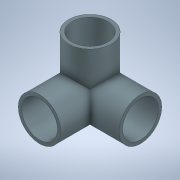
# Autodesk Inventor part: hoek drieweg
Saved by Autodesk Inventor 2020.2 (Build 242310000, 310)
## iProperties
Created: 2019-11-27
Part Number: hoek drieweg
Material: ABS Plastic
Document SubType Name: Modeling
Designer: Gebruiker
Density: 1.06 g/cm^3
Appearance: Lead
Author: Gebruiker
Autodesk Inventor part; units mm, degrees
sketch "Sketch1" plane through (0, 0, 0) normal (0, 1, 0) x (-1, 0, 0)
  line L0 (0, 0) -> (0, 30)
  line L1 (0, 0) -> (-30, 0)
  dimension "d0" = 30
  dimension "d1" = 30
  constraints: 4 end point, 1 horizontal, 1 vertical
  measures "d0" distance of L0.start L0.end
  measures "d1" distance of L0.start L1.end
ref_plane "Work Plane1" through (0, 0, 30) normal (0, 0, 1) x (1, 0, 0)
sketch "Sketch2" plane through (0, 0, 30) normal (0, 0, 1) x (1, 0, 0)
  circle A0 centre (0, 0) radius 12.65
  dimension "d2" = 25.3
  constraints: 1 centre point, 1 coincident
  measures "d2" diameter of A0
sketch "Sketch3" plane through (0, 0, 0) normal (0, 1, 0) x (-1, 0, 0)
  line L0 (0, 0) -> (0, 30) projected
sweep "Sweep1" add profiles "Sketch2" path "Sketch3"
sketch "Sketch4" plane through (0, 0, 0) normal (1, 0, 0) x (0, 1, 0)
  line L0 (0, 0) -> (30, 0)
  dimension "d5" = 30
  constraints: 2 end point, 1 horizontal
  measures "d5" distance of L0.start L0.end
ref_plane "Work Plane2" through (0, 30, 0) normal (0, 1, 0) x (-1, 0, 0)
sketch "Sketch5" plane through (0, 30, 0) normal (0, 1, 0) x (-1, 0, 0)
  circle A0 centre (0, 0) radius 12.65
  dimension "d6" = 25.3
  constraints: 1 centre point, 1 coincident
  measures "d6" diameter of A0
sweep "Sweep2" add profiles "Sketch5" path "Sketch4" separate body
sketch "Sketch6" plane through (0, 0, 0) normal (0, 1, 0) x (-1, 0, 0)
  line L0 (0, 0) -> (-30, 0) projected
ref_plane "Work Plane3" through (30, 0, 0) normal (1, 0, 0) x (0, 1, 0)
sketch "Sketch7" plane through (30, 0, 0) normal (1, 0, 0) x (0, 1, 0)
  circle A0 centre (0, 0) radius 12.65
  dimension "d9" = 25.3
  constraints: 1 centre point, 1 coincident
  measures "d9" diameter of A0
sweep "Sweep3" add profiles "Sketch7" path "Sketch6" separate body
sketch "Sketch8" plane through (0, 0, 0) normal (-1, 0, 0) x (0, 0, 1)
  circle A0 centre (0, 0) radius 12.65 projected
  line L0 (-12.65, 0) -> (12.65, 0) projected
  line L1 (0, 12.65) -> (0, -12.65) projected
sketch "Sketch10" plane through (0, 0, 0) normal (0, -1, 0) x (1, 0, 0)
  circle A0 centre (0, 0) radius 12.65 projected
sketch3d "3D Sketch1"
  arc A0 (-12.65, 0, 0) -> (0, 0, -12.65) centre (0, 0, 0) ccw
  arc A1 (0, 0, -12.65) -> (12.65, 0, 0) centre (0, 0, 0) ccw
  arc A2 (12.65, 0, 0) -> (0, 0, 12.65) centre (0, 0, 0) ccw
  arc A3 (0, 0, 12.65) -> (-12.65, 0, 0) centre (0, 0, 0) ccw
sweep "Sweep4" add profiles "Sketch8" path "3D Sketch1" separate body picked at (-0.9383, -8.3276) contours A0 L0 L1
sketch "Sketch12" plane through (0, 30, 0) normal (0, 1, 0) x (1, 0, 0)
  circle A0 centre (0, 0) radius 10.65
  dimension "d16" = 21.3
  constraints: 1 centre point, 1 coincident
  measures "d16" diameter of A0
extrude "Extrusion1" cut sketch "Sketch12" against normal blind 15 bodies 2
sketch "Sketch13" plane through (30, 0, 0) normal (1, 0, 0) x (0, 0, -1)
  circle A0 centre (0, 0) radius 10.65
  dimension "d19" = 21.3
  constraints: 1 centre point, 1 coincident
  measures "d19" diameter of A0
extrude "Extrusion2" cut sketch "Sketch13" against normal blind 15 bodies 3
sketch "Sketch14" plane through (0, 0, 30) normal (0, 0, 1) x (1, 0, 0)
  circle A0 centre (0, 0) radius 10.65
  dimension "d22" = 21.3
  constraints: 1 centre point, 1 coincident
  measures "d22" diameter of A0
extrude "Extrusion3" cut sketch "Sketch14" against normal blind 15 bodies 1
equation "\"d1\" = d0"
body "Solid1"
body "Solid2"
body "Solid3"
body "Solid4"
